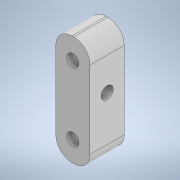
# Autodesk Inventor part: Slider7
Saved by Autodesk Inventor 2022 (Build 260153000, 153)
## iProperties
Created: 2022-01-25
Part Number: Slider7
Material: Generic
Document SubType Name: Modeling
Designer: songy
Density: 1 g/cm^3
Appearance: Default
Author: songy
Autodesk Inventor part; units mm, degrees
ref_plane "YZ Plane" through (0, 0, 0) normal (1, 0, 0) x (0, 1, 0)
ref_plane "XZ Plane" through (0, 0, 0) normal (0, 1, 0) x (-1, 0, 0)
ref_plane "XY Plane" through (0, 0, 0) normal (0, 0, 1) x (1, 0, 0)
sketch "Sketch1" plane through (0, 0, 0) normal (0, 0, 1) x (1, 0, 0)
  line L0 (0, 0) -> (12.7, 0)
  line L1 (12.7, 0) -> (12.7, 50.8)
  line L2 (12.7, 50.8) -> (0, 50.8)
  line L3 (0, 50.8) -> (0, 0)
  dimension "d0" = 12.7
  dimension "d1" = 50.8
  constraints: 8 end point, 2 parallel, 1 horizontal, 1 perpendicular
  measures "d0" distance between parallel lines of L1 L3
  measures "d1" distance between parallel lines of L0 L2
extrude "Extrusion1" add sketch "Sketch1" along normal blind 12.7
sketch "Sketch5" plane through (0, 0, 12.7) normal (0, 0, 1) x (1, 0, 0)
  line L0 (12.7, 0) -> (12.7, 50.8) projected
  line L1 (12.7, 50.8) -> (0, 50.8) projected
  line L2 (0, 0) -> (12.7, 0) projected
  point P0 (6.35, 38.1)
  point P1 (6.35, 12.7)
  point P2 (6.35, 50.8)
  dimension "d19" = 6.35
  dimension "d20" = 12.7
  dimension "d21" = 6.35
  dimension "d22" = 12.7
  constraints: 1 midpoint
  measures "d19" distance from line of L0 point (6.35, 38.1)
  measures "d20" distance of point (6.35, 50.8) point (6.35, 38.1)
  measures "d21" distance from line of L0 point (6.35, 12.7)
  measures "d22" distance from line of L2 point (6.35, 12.7)
hole "Hole1" at (6.35, 38.1, 12.7) at (6.35, 12.7, 12.7) direction (0, 0, -1) diameter 4.5 end through all clearance for "Flat Head Machine Screw" size "M4" standard "Ansi Metric M Profile"
sketch "Sketch6" plane through (0, 0, 12.7) normal (0, 0, 1) x (1, 0, 0)
  line L0 (12.7, 50.8) -> (0, 50.8) projected
  line L1 (0, 50.8) -> (0, 45.8)
  line L2 (0, 50.8) -> (0, 0) projected
  line L3 (12.7, 0) -> (12.7, 50.8) projected
  line L4 (12.7, 45.8) -> (12.7, 50.8)
  line L5 (12.7, 50.8) -> (0, 50.8)
  line L6 (0, 45.8) -> (12.7, 45.8)
  dimension "d32" = 5
  constraints: 8 end point, 2 point on line, 1 collinear, 1 parallel, 1 perpendicular
  measures "d32" distance of L0.end L1.end
extrude "Extrusion4" cut sketch "Sketch6" against normal blind 12.7
sketch "Sketch7" plane through (0, 0, 12.7) normal (0, 0, 1) x (1, 0, 0)
  line L0 (0, 45.8) -> (0, 0) projected
  line L1 (0, 0) -> (0, 5)
  line L2 (12.7, 0) -> (12.7, 45.8) projected
  line L3 (12.7, 5) -> (12.7, 0)
  line L4 (0, 0) -> (12.7, 0) projected
  line L5 (12.7, 0) -> (0, 0)
  line L6 (0, 5) -> (12.7, 5)
  dimension "d35" = 5
  constraints: 8 end point, 2 collinear, 2 point on line, 1 perpendicular
  measures "d35" distance of L0.end L1.end
extrude "Extrusion5" cut sketch "Sketch7" against normal blind 12.7
fillet "Fillet3" radius 6 2 edges at (12.7, 45.8, 6.35) (0, 45.8, 6.35)
fillet "Fillet4" radius 6 2 edges at (12.7, 5, 6.35) (0, 5, 6.35)
sketch "Sketch8" plane through (12.7, 39.8, 12.7) normal (1, 0, 0) x (0, 0, -1)
  circle A0 centre (6.35, -12.044) radius 2.25
  line L0 (12.7, -28.8) -> (12.7, 0) projected
  line L1 (12.7, -28.8) -> (0, -28.8) projected
  line L2 (0, -34.8) -> (12.7, -34.8) projected
  point P0 (12.7, -39.8)
  dimension "d43" = 6.35
  dimension "d44" = 4.5
  dimension "d49" = 16.756
  constraints: 1 centre point
  measures "d43" distance from line of L0 A0.centre
  measures "d44" diameter of A0
  measures "d49" distance from line of L1 A0.centre
extrude "Extrusion6" cut sketch "Sketch8" against normal blind 12.7
body "Solid1"
